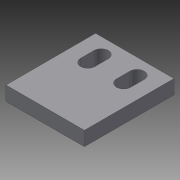
# Autodesk Inventor part: Air2D_Hinge_Top
Saved by Autodesk Inventor 2014 (Build 180170000, 170)
## iProperties
Created: 2014-09-30
Part Number: Air2D_Hinge_Top
Material: Generic
Document SubType Name: Modeling
Designer: ThatOtherGuy
Density: 1 g/cm^3
Appearance: Default
Author: ThatOtherGuy
Autodesk Inventor part; units mm, degrees
ref_plane "YZ Plane" through (0, 0, 0) normal (1, 0, 0) x (0, 1, 0)
ref_plane "XZ Plane" through (0, 0, 0) normal (0, 1, 0) x (-1, 0, 0)
ref_plane "XY Plane" through (0, 0, 0) normal (0, 0, 1) x (1, 0, 0)
sketch "Sketch1" plane through (0, 0, 0) normal (0, 0, 1) x (1, 0, 0)
  line L0 (0, 0) -> (0, 12.5)
  line L1 (0, 12.5) -> (8.75, 12.5)
  line L2 (8.75, 12.5) -> (8.75, 0)
  line L3 (8.75, 0) -> (0, 0)
  line L4 (3.5, 7.25) -> (3.5, 5.25) construction
  line L5 (1.9, 7.25) -> (1.9, 5.25)
  line L6 (5.1, 5.25) -> (5.1, 7.25)
  arc A0 (5.1, 7.25) -> (1.9, 7.25) centre (3.5, 7.25) ccw
  arc A1 (1.9, 5.25) -> (5.1, 5.25) centre (3.5, 5.25) ccw
  point P0 (3.5, 6.25)
  dimension "d13" = 3.2
  dimension "d14" = 2
  dimension "d15" = 6.25
  dimension "d17" = 12.5
  dimension "d18" = 8.75
  dimension "d19" = 3.5
  constraints: 16 end point, 4 parallel, 4 point on circle, 4 tangent, 2 centre point, 1 midpoint, 1 perpendicular, 1 vertical
  measures "d13" distance between parallel lines of L5 L6
  measures "d14" distance of L4.start L4.end
  measures "d15" distance from line of L1 point (3.5, 6.25)
  measures "d17" distance of L0.start L0.end
  measures "d18" distance of L0.end L1.end
  measures "d19" distance from line of L0 point (3.5, 6.25)
extrude "Extrusion1" add sketch "Sketch1" along normal blind 3.175
mirror "Mirror1" about plane through (0, 12.5, 0) normal (-1, 0, 0) of "Extrusion1"
equation "\"d15\" = 0.5 * d17"
equation "\"d8\" = THICKA"
equation "\"THICKA\" = 3.175"
equation "\"THICKB\" = 6.731"
equation "\"THICKC\" = 12.7"
equation "\"MAGDIA\" = 9.5"
equation "\"BALLDIA\" = 12"
body "Solid1"
